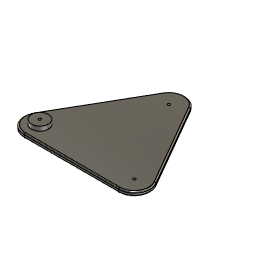
amrest_A (Autodesk Fusion 360 design; units mm, degrees)
Autodesk Fusion 360 part; units mm, degrees
sketch "スケッチ1" plane through (0, 0, 0) normal (0, 0, 1) x (1, 0, 0)
  circle A0 centre (0, 0) radius 13.85
  circle A1 centre (0, 0) radius 25
  line L0 (0, 25) -> (110, 25)
  line L1 (110, 25) -> (110, -25)
  line L2 (110, -25) -> (0, -25)
  line L3 (110, 25) -> (128, 25)
  line L4 (128, 25) -> (128, -25)
  line L5 (128, -25) -> (110, -25)
  line L6 (110, -25) -> (110, 25)
  circle A2 centre (0, -120) radius 13.95
  circle A3 centre (0, -120) radius 25
  line L7 (150, 145) -> (150, 95)
  circle A4 centre (0, 120) radius 13.75
  line L8 (0, 145) -> (150, 145)
  line L9 (150, 95) -> (0, 95)
  line L10 (150, 95) -> (150, 145)
  circle A5 centre (0, 120) radius 25
  circle A6 centre (150, 120) radius 25
  circle A7 centre (150, 120) radius 13.75
  circle A8 centre (0, 250) radius 2
  circle A9 centre (0, 250) radius 25
  circle A10 centre (100, 250) radius 25
  circle A11 centre (100, 250) radius 13.5
  line L11 (100, 275) -> (250, 275)
  line L12 (250, 275) -> (250, 225)
  line L13 (250, 225) -> (100, 225)
  line L14 (100, 225) -> (100, 275)
  circle A12 centre (250, 250) radius 25
  circle A13 centre (250, 250) radius 2
  line L15 (100, 250) -> (175, 379.9038)
  line L16 (100, 250) -> (250, 250) construction
  line L17 (175, 379.9038) -> (250, 250)
  circle A14 centre (175, 379.9038) radius 25
  line L18 (100, 250) -> (175, 379.9038)
  line L19 (78.3494, 262.5) -> (153.3494, 392.4038)
  line L20 (196.6506, 392.4038) -> (271.6506, 262.5)
  circle A15 centre (175, 379.9038) radius 2
  circle A16 centre (100, 250) radius 2
  point P0 (0, 120)
  dimension "d1" = 27.7
  dimension "d2" = 50
  dimension "d3" = 110
  dimension "d4" = 18
  dimension "d26" = 27.9
  dimension "d27" = 50
  dimension "d37" = 27.5
  dimension "d38" = 50
  dimension "d39" = 150
  dimension "d41" = 50
  dimension "d42" = 27.5
  dimension "d45" = 4
  dimension "d46" = 50
  dimension "d49" = 50
  dimension "d50" = 27
  dimension "d51" = 150
  dimension "d52" = 50
  dimension "d53" = 4
  dimension "d54" = 60
  dimension "d55" = 150
  dimension "d56" = 50
  dimension "d57" = 150
  dimension "d59" = 4
  dimension "d64" = 4
  constraint coincident A0.centre A1.centre
  constraint coincident A1 L0.start
  constraint horizontal L0
  constraint perpendicular L0 L1
  constraint coincident A1 L2.end
  constraint tangent A1 L2
  constraint perpendicular L1 L2
  constraint horizontal L3
  constraint vertical L4
  constraint horizontal L5
  constraint vertical L6
  constraint concentric A2 A3
  constraint coincident P0 A4.centre
  constraint coincident L8.start A5
  constraint horizontal L8
  constraint perpendicular L7 L8
  constraint coincident L9.end A5
  constraint tangent L9 A5
  constraint perpendicular L7 L9
  constraint vertical L10
  constraint midpoint L10 A6.centre
  constraint concentric A6 A7
  constraint concentric A8 A9
  constraint concentric A10 A11
  constraint horizontal L11
  constraint vertical L12
  constraint horizontal L13
  constraint vertical L14
  constraint coincident A10 L11.start
  constraint midpoint L12 A12.centre
  constraint concentric A12 A13
  constraint horizontal L16
  constraint coincident A10.centre A11.centre
  constraint coincident L15.end L17.start
  constraint parallel L15 L19
  constraint parallel L17 L20
  constraint coincident A14 L19.end
  constraint coincident A14 L20.start
  constraint concentric A14 A15
  constraint concentric A11 A16
  measures "d1" diameter of A0
  measures "d2" diameter of A1
  measures "d3" distance of L0.start L0.end
  measures "d4" distance of L0.end L3.end
  measures "d26" diameter of A2
  measures "d27" diameter of A3
  measures "d37" diameter of A4
  measures "d38" diameter of A5
  measures "d39" distance of L8.start L7.start
  measures "d41" diameter of A6
  measures "d42" diameter of A7
  measures "d45" diameter of A8
  measures "d46" diameter of A9
  measures "d49" diameter of A10
  measures "d50" diameter of A11
  measures "d51" distance of L11.start L11.end
  measures "d52" diameter of A12
  measures "d53" diameter of A13
  measures "d54" angle of L15 L16
  measures "d55" distance of A10.centre L15.end
  measures "d56" diameter of A14
  measures "d57" distance of L15.end A10.centre
  measures "d59" diameter of A15
  measures "d64" diameter of A16
extrude "押し出し1" add sketch "スケッチ1" along normal blind 7 contours A1 | A1 L0 L1 L2 L6 makes body 1
extrude "押し出し2" add sketch "スケッチ1" along normal blind 7 contours L1 L3 L4 L5 L6 bodies 1
extrude "押し出し3" add sketch "スケッチ1" against normal blind 10 contours L1 L3 L4 L5 L6 bodies 1
sketch "スケッチ2" plane through (0, 0, -10) normal (0, 0, -1) x (1, 0, 0)
  line L0 (128, 25) -> (110, 25)
  line L1 (110, 25) -> (110, -25)
  line L2 (110, -25) -> (128, -25)
  line L3 (128, -25) -> (128, 25)
  line L4 (128, 25) -> (160, 25)
  line L5 (160, 25) -> (160, -25)
  line L6 (160, -25) -> (128, -25)
  line L7 (128, -25) -> (128, 25)
  circle A0 centre (160, 0) radius 25
  circle A1 centre (160, 0) radius 13.75
  circle A2 centre (160, 0) radius 1.6
  circle A3 centre (160, 80) radius 25
  circle A4 centre (160, 80) radius 1.6
  dimension "d11" = 32
  dimension "d12" = 50
  dimension "d13" = 50
  dimension "d14" = 27.5
  dimension "d19" = 3.2
  dimension "d22" = 50
  dimension "d23" = 3.2
  constraint horizontal L4
  constraint vertical L5
  constraint horizontal L6
  constraint vertical L7
  constraint coincident L0.start L3.end
  constraint midpoint L5 A0.centre
  constraint concentric A0 A1
  constraint concentric A0 A2
  constraint concentric A3 A4
  measures "d11" distance of L0.start L4.end
  measures "d12" distance of L0.start L2.end
  measures "d13" diameter of A0
  measures "d14" diameter of A1
  measures "d19" diameter of A2
  measures "d22" diameter of A3
  measures "d23" diameter of A4
extrude "押し出し4" add sketch "スケッチ2" against normal blind 10 contours L3 L4 L6 L7 A0 | L5 A0 A1 | L5 A0 A1 bodies 1
extrude "押し出し5" add sketch "スケッチ2" against normal blind 20 contours L5 A1 A2 | L5 A1 A2 | L5 A2 | L5 A2 bodies 1
extrude "押し出し6" cut sketch "スケッチ2" along normal mid plane 100 contours L5 A2 | L5 A2 bodies 1
extrude "押し出し7" add sketch "スケッチ2" along normal blind 5 separate body contours A3 makes body 2
extrude "押し出し8" add sketch "スケッチ1" along normal blind 10 separate body contours A3 makes body 3
sketch "スケッチ3" plane through (0, 0, -10) normal (0, 0, -1) x (1, 0, 0)
  circle A0 centre (160, 80) radius 3
  dimension "d30" = 6
  measures "d30" diameter of A0
extrude "押し出し9" cut sketch "スケッチ3" along normal blind 2 bodies 2
extrude "押し出し10" add sketch "スケッチ1" along normal blind 7 separate body contours L7 L10 A6 A7 | L8 L9 A5 A6 | L7 L10 A6 A7 | A5 makes body 4
extrude "押し出し11" add sketch "スケッチ1" along normal blind 4 separate body contours A9 makes body 5
extrude "押し出し12" add sketch "スケッチ1" along normal blind 7 separate body contours A10 A11 L14 | A10 L11 L15 L18 | A10 L11 L15 A14 L18 L19 | A10 A11 L14 L15 L18 | A10 L11 L13 A12 L15 L17 L18 | A10 A11 L14 L15 L18 | L11 L15 L17 A14 L18 | A11 L14 A16 | A11 L14 L15 L18 A16 | L15 L17 A14 L18 A15 | A11 L14 L15 L18 A16 | L11 A12 L17 A14 L20 | L11 A12 L17 | L15 L17 A14 L18 A15 | L14 L15 L18 A16 | L14 A16 | L12 A12 A13 L17 | L12 A12 A13 | L14 L15 L18 A16 | L12 A12 A13 L17 makes body 6
extrude "押し出し13" add sketch "スケッチ1" along normal blind 14 contours A11 L14 A16 | A11 L14 L15 L18 A16 | A11 L14 L15 L18 A16 | L14 L15 L18 A16 | L14 A16 | L14 L15 L18 A16 bodies 6
extrude "押し出し14" cut sketch "スケッチ1" along normal blind 30 contours L14 L15 L18 A16 | L14 A16 | L14 L15 L18 A16 bodies 6
fillet "フィレット3" radius 2 1 edges at (-23.3082, 240.9596, 4) on bodies 5
fillet "フィレット4" radius 2 8 edges at (75, 95, 7) (175, 120, 7) (75, 145, 7) (-25, 120, 7) (-25, 120, 0) (75, 145, 0) (175, 120, 0) (75, 95, 0) on bodies 4
fillet "フィレット5" radius 2 6 faces at (103.3494, 305.8013, 4.6667) (77.7532, 261.4053, 4.6667) (200, 225, 2.3333) (263.0359, 228.6677, 2.3333) (221.6506, 349.1025, 2.3333) (195.2985, 394.4974, 2.3333) on bodies 6
hidden bodies 1 2 3 4 5
